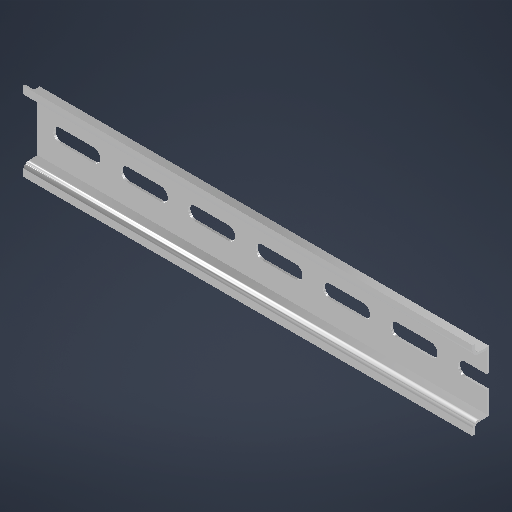
# Autodesk Inventor part: din_rail
Saved by Autodesk Inventor 2025 (Build 290162000, 162)
## iProperties
Created: 2024-08-31
Part Number: din_rail
Material: Aluminum 6061
Document SubType Name: Modeling
Designer: Dawid
Density: 2.7 g/cm^3
Appearance: Aluminum - Flat
Author: Dawid
Autodesk Inventor part; units mm, degrees
ref_plane "YZ Plane" through (0, 0, 0) normal (1, 0, 0) x (0, 1, 0)
ref_plane "XZ Plane" through (0, 0, 0) normal (0, 1, 0) x (-1, 0, 0)
ref_plane "XY Plane" through (0, 0, 0) normal (0, 0, 1) x (1, 0, 0)
sketch "Sketch1" plane through (0, 0, 0) normal (1, 0, 0) x (0, 1, 0)
  line L0 (12.5, 0) -> (-12.5, 0)
  line L1 (12.5, 0) -> (12.5, 3.5)
  line L2 (15.5, 6.5) -> (17.5, 6.5)
  line L3 (-12.5, 0) -> (-12.5, 3.5)
  line L4 (-15.5, 6.5) -> (-17.5, 6.5)
  line L5 (17.5, 5.5) -> (15.5, 5.5)
  line L6 (13.5, 3.5) -> (13.5, -1)
  line L7 (13.5, -1) -> (-13.5, -1)
  line L8 (-13.5, -1) -> (-13.5, 3.5)
  line L9 (-15.5, 5.5) -> (-17.5, 5.5)
  line L10 (17.5, 5.5) -> (17.5, 6.5)
  line L11 (-17.5, 5.5) -> (-17.5, 6.5)
  arc A0 (15.5, 5.5) -> (13.5, 3.5) centre (15.5, 3.5) ccw
  arc A1 (15.5, 6.5) -> (12.5, 3.5) centre (15.5, 3.5) ccw
  arc A2 (-12.5, 3.5) -> (-15.5, 6.5) centre (-15.5, 3.5) ccw
  arc A3 (-13.5, 3.5) -> (-15.5, 5.5) centre (-15.5, 3.5) ccw
  point P0 (0, 0)
  point P1 (0, 0)
  dimension "d0" = 25
  dimension "d2" = 1
  dimension "d3" = 35
  dimension "d4" = 2
  dimension "d5" = 2
  dimension "d6" = 7.5
  constraints: 24 end point, 8 point on circle, 8 tangent, 4 centre point, 4 perpendicular, 3 coincident, 3 vertical, 1 collinear, 1 horizontal, 1 horizontal alignment, 1 midpoint, 1 parallel, 4 other
  measures "d0" distance between parallel lines of L3 L1
  measures "d2" distance between parallel lines of L2 L5
  measures "d3" distance of L4.end L2.end
  measures "d4" radius of A0
  measures "d5" radius of A3
  measures "d6" distance between parallel lines of L7 L4
extrude "Extrusion1" add sketch "Sketch1" along normal blind 200
sketch "Sketch2" plane through (0, -12.5, 0) normal (0, 0, 1) x (1, 0, 0)
  line L0 (10, 12.5) -> (25, 12.5) construction
  line L1 (10, 9.5) -> (25, 9.5)
  line L2 (25, 15.5) -> (10, 15.5)
  arc A0 (10, 15.5) -> (10, 9.5) centre (10, 12.5) ccw
  arc A1 (25, 9.5) -> (25, 15.5) centre (25, 12.5) ccw
  line L3 (0, 25) -> (0, 0) projected
  point P0 (0, 12.5)
  point P1 (17.5, 12.5)
  point P2 (0, 12.5)
  dimension "d9" = 15
  dimension "d10" = 6
  dimension "d11" = 10
  constraints: 8 end point, 4 point on circle, 4 tangent, 2 centre point, 2 midpoint, 1 horizontal, 1 parallel
  measures "d9" distance of L0.start L0.end
  measures "d10" distance between parallel lines of L2 L1
  measures "d11" distance of point (0, 12.5) L0.start
extrude "Extrusion2" cut sketch "Sketch2" against normal through all
pattern_linear "Rectangular Pattern1" count 10 spacing 30 along (1, 0, 0) of "Extrusion2"
equation "\"d12\" = d9"
body "Solid1"
